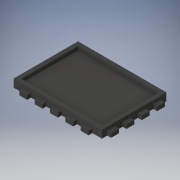
# Autodesk Inventor part: bottom
Saved by Autodesk Inventor 2019 (Build 230136000, 136)
## iProperties
Created: 2018-06-07
Part Number: bottom
Material: PBT Plastic Black
Document SubType Name: Modeling
Designer: stra92745
Density: 1.31 g/cm^3
Appearance: Smooth - White
Author: stra92745
Autodesk Inventor part; units mm, degrees
ref_plane "YZ Plane" through (0, 0, 0) normal (1, 0, 0) x (0, 1, 0)
ref_plane "XZ Plane" through (0, 0, 0) normal (0, 1, 0) x (-1, 0, 0)
ref_plane "XY Plane" through (0, 0, 0) normal (0, 0, 1) x (1, 0, 0)
sketch "Sketch1" plane through (0, 0, 0) normal (0, 1, 0) x (-1, 0, 0)
  line L0 (0, 0) -> (-100, 0)
  line L1 (-100, 0) -> (-100, -75)
  line L2 (-100, -75) -> (0, -75)
  line L3 (0, -75) -> (0, 0)
  dimension "d0" = 100
  dimension "d1" = 75
  constraints: 8 end point, 2 parallel, 1 horizontal, 1 perpendicular
  measures "d0" distance of L2.end L1.end
  measures "d1" distance of L1.end L0.end
extrude "Extrusion1" add sketch "Sketch1" along normal blind 4
sketch "Sketch2" plane through (0, 4, 0) normal (0, 1, 0) x (1, 0, 0)
  line L0 (0, 0) -> (100, 0) construction
  line L1 (100, 0) -> (100, 75) construction
  line L2 (100, 75) -> (0, 75) construction
  line L3 (0, 75) -> (0, 0) construction
  line L4 (4, 71) -> (96, 71)
  line L5 (96, 71) -> (96, 4)
  line L6 (96, 4) -> (4, 4)
  line L7 (4, 4) -> (4, 71)
  line L8 (92, 67) -> (8, 67)
  line L9 (8, 67) -> (8, 8)
  line L10 (8, 8) -> (92, 8)
  line L11 (92, 8) -> (92, 67)
  dimension "d4" = 4
  dimension "d5" = 4
  constraints: 16 end point, 6 other
  measures "d4" distance between parallel lines of L2 L4
  measures "d5" distance between parallel lines of L4 L8
extrude "Extrusion2" add sketch "Sketch2" along normal blind 4
sketch "Sketch3" plane through (0, 4, 0) normal (0, 1, 0) x (1, 0, 0)
  line L0 (100, 75) -> (0, 75) construction
  line L1 (0, 75) -> (0, 0) construction
  line L2 (0, 0) -> (100, 0) construction
  line L3 (100, 0) -> (100, 75) construction
  line L4 (4, 71) -> (96, 71) construction
  line L5 (96, 71) -> (96, 4) construction
  line L6 (96, 4) -> (4, 4) construction
  line L7 (4, 4) -> (4, 71) construction
  line L8 (0, 37.5) -> (100, 37.5) construction
  line L9 (50, 75) -> (50, 0) construction
  line L10 (0, 65.5) -> (4, 65.5)
  line L11 (4, 65.5) -> (4, 71)
  line L12 (4, 71) -> (14, 71)
  line L13 (4, 71) -> (96, 71) projected
  line L14 (14, 71) -> (14, 75)
  line L15 (14, 75) -> (0, 75)
  line L16 (0, 75) -> (0, 65.5)
  line L17 (0, 57.5) -> (4, 57.5)
  line L18 (4, 57.5) -> (4, 49.5)
  line L19 (4, 71) -> (4, 4) projected
  line L20 (4, 49.5) -> (0, 49.5)
  line L21 (0, 49.5) -> (0, 57.5)
  line L22 (0, 41.5) -> (4, 41.5)
  line L23 (4, 37.5) -> (4, 41.5)
  line L24 (0, 41.5) -> (0, 37.5)
  line L25 (22, 75) -> (22, 71)
  line L26 (22, 71) -> (30, 71)
  line L27 (30, 71) -> (30, 75)
  line L28 (30, 75) -> (22, 75)
  line L29 (38, 75) -> (38, 71)
  line L30 (38, 71) -> (46, 71)
  line L31 (46, 71) -> (46, 75)
  line L32 (46, 75) -> (38, 75)
  line L33 (0, 9.5) -> (4, 9.5)
  line L34 (4, 9.5) -> (4, 4)
  line L35 (4, 4) -> (14, 4)
  line L36 (14, 4) -> (14, 0)
  line L37 (14, 0) -> (0, 0)
  line L38 (0, 0) -> (0, 9.5)
  line L39 (0, 17.5) -> (4, 17.5)
  line L40 (4, 17.5) -> (4, 25.5)
  line L41 (4, 25.5) -> (0, 25.5)
  line L42 (0, 25.5) -> (0, 17.5)
  line L43 (0, 33.5) -> (4, 33.5)
  line L44 (4, 37.5) -> (4, 33.5)
  line L45 (0, 33.5) -> (0, 37.5)
  line L46 (22, 0) -> (22, 4)
  line L47 (22, 4) -> (30, 4)
  line L48 (30, 4) -> (30, 0)
  line L49 (30, 0) -> (22, 0)
  line L50 (38, 0) -> (38, 4)
  line L51 (38, 4) -> (46, 4)
  line L52 (46, 4) -> (46, 0)
  line L53 (46, 0) -> (38, 0)
  line L54 (100, 75) -> (100, 0) construction
  line L55 (96, 4) -> (96, 71) construction
  line L56 (100, 65.5) -> (96, 65.5)
  line L57 (96, 65.5) -> (96, 71)
  line L58 (96, 71) -> (86, 71)
  line L59 (86, 71) -> (86, 75)
  line L60 (86, 75) -> (100, 75)
  line L61 (100, 75) -> (100, 65.5)
  line L62 (100, 57.5) -> (96, 57.5)
  line L63 (96, 57.5) -> (96, 49.5)
  line L64 (96, 71) -> (96, 4)
  line L65 (96, 49.5) -> (100, 49.5)
  line L66 (100, 49.5) -> (100, 57.5)
  line L67 (100, 41.5) -> (96, 41.5)
  line L68 (96, 37.5) -> (96, 41.5)
  line L69 (100, 41.5) -> (100, 37.5)
  line L70 (78, 75) -> (78, 71)
  line L71 (78, 71) -> (70, 71)
  line L72 (70, 71) -> (70, 75)
  line L73 (70, 75) -> (78, 75)
  line L74 (62, 75) -> (62, 71)
  line L75 (62, 71) -> (54, 71)
  line L76 (54, 71) -> (54, 75)
  line L77 (54, 75) -> (62, 75)
  line L78 (78, 0) -> (78, 4)
  line L79 (70, 4) -> (70, 0)
  line L80 (78, 4) -> (70, 4)
  line L81 (70, 0) -> (78, 0)
  line L82 (54, 4) -> (54, 0)
  line L83 (62, 4) -> (54, 4)
  line L84 (54, 0) -> (62, 0)
  line L85 (62, 0) -> (62, 4)
  line L86 (96, 4) -> (86, 4)
  line L87 (100, 9.5) -> (96, 9.5)
  line L88 (96, 9.5) -> (96, 4)
  line L89 (86, 4) -> (86, 0)
  line L90 (86, 0) -> (100, 0)
  line L91 (96, 17.5) -> (96, 25.5)
  line L92 (100, 17.5) -> (96, 17.5)
  line L93 (96, 25.5) -> (100, 25.5)
  line L94 (96, 37.5) -> (96, 33.5)
  line L95 (100, 33.5) -> (96, 33.5)
  line L96 (100, 33.5) -> (100, 37.5)
  line L97 (100, 25.5) -> (100, 17.5)
  line L98 (100, 0) -> (100, 9.5)
  dimension "d9" = 8
  dimension "d11" = 4
  dimension "d12" = 8
  dimension "d13" = 8
  dimension "d14" = 8
  dimension "d15" = 8
  dimension "d16" = 8
  dimension "d17" = 4
  dimension "d18" = 8
  constraints: 186 end point, 55 symmetric about line, 26 point on line, 9 perpendicular, 6 collinear, 5 midpoint, 1 vertical, 3 other
  measures "d9" distance between parallel lines of L17 L10
  measures "d11" distance between parallel lines of L8 L22
  measures "d12" distance between parallel lines of L22 L20
  measures "d13" distance between parallel lines of L17 L20
  measures "d14" distance of L27.end L25.start
  measures "d15" distance between parallel lines of L27 L29
  measures "d16" distance of L31.end L29.start
  measures "d17" distance between parallel lines of L9 L31
  measures "d18" distance between parallel lines of L14 L25
extrude "Extrusion3" cut sketch "Sketch3" against normal up to surface (4 mm away)
body "Solid1"
